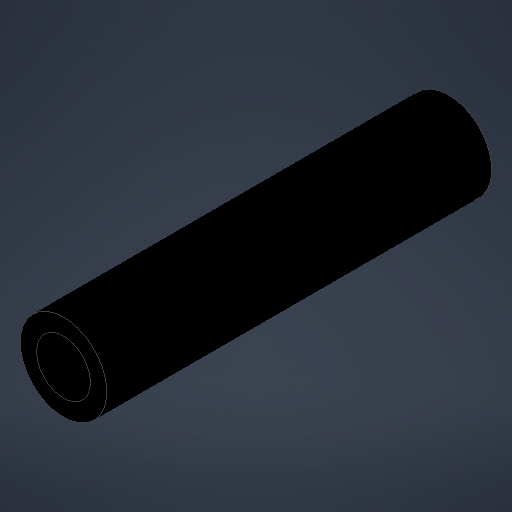
# Autodesk Inventor part: Rod Housing Jetson
Saved by Autodesk Inventor 2026.1 (Build 301233020, 233B)
## iProperties
Created: 2026-02-20
Part Number: Rod Housing Jetson
Material: Generic
Document SubType Name: Modeling
Designer: Bahaa
Density: 1 g/cm^3
Appearance: Default
Author: Bahaa
Autodesk Inventor part; units mm, degrees
ref_plane "YZ Plane" through (0, 0, 0) normal (1, 0, 0) x (0, 1, 0)
ref_plane "XZ Plane" through (0, 0, 0) normal (0, 1, 0) x (-1, 0, 0)
ref_plane "XY Plane" through (0, 0, 0) normal (0, 0, 1) x (1, 0, 0)
sketch "Sketch1" plane through (0, 0, 0) normal (0, 1, 0) x (-1, 0, 0)
  circle A0 centre (0, 0) radius 2.25
  circle A1 centre (0, 0) radius 1.4
  dimension "d0" = 4.5
  dimension "d1" = 2.8
  constraints: 2 centre point, 2 coincident
  measures "d0" diameter of A0
  measures "d1" diameter of A1
extrude "Extrusion1" add sketch "Sketch1" along normal blind 20
body "Solid1"
